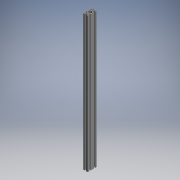
# Autodesk Inventor part: HFS5-2040-600-Z5-YA10-YB590
Saved by Autodesk Inventor 2017.3 (Build 213256000, 256)
## iProperties
Part Number: HFS5-2040-600-Z5-YA10-YB590
Material: Generic
Catalog Web Link: www.cadenas.de
Description: NFS5-2040, NFSB5-2040, HFS5-2040, HFSB5-2040, CAF5-2040, NFSF5-2040, HFSF5-2040-HFS5 Series Aluminum Extrusions 20,40 Square -2 Slots-
Vendor: MISUMI
Document SubType Name: Modeling
Designer: partserver
Manufacturer: MISUMI
Mass: 193.574 g
Surface Area: 1890.72 cm^2
Volume: 193.574 cm^3
Density: 1 g/cm^3
Appearance: PSOLRGB-175-175-175
Category: PARTsolutions
Company: MISUMI
Title: HFS5-2040-600-Z5-YA10-YB590
Author: Cadenas PARTsolutions
Comments: HFS5 Series Aluminum Extrusions 20,40 Square -2 Slots-
PSOL_IDENT_0: {$CADENAS_DATA\23d-libs\misumi\metric\38_al_extrusions_blackets\5\hfs5_2040.prj},643 {VTYP=3D},{NB=H
PSOL_IDENT_1: FS5-2040-600-Z5-YA10-YB590},{LINA=HFS5-2040-600-Z5-YA10-YB590},{NN=NFS5-2040, NFSB5-2040, HFS5-2040,
PSOL_IDENT_2: HFSB5-2040, CAF5-2040, NFSF5-2040, HFSF5-2040},{DATE=09.09.2019 15:28:27},{GEOMDATE=28.10.2014 00:0
PSOL_IDENT_3: 0:00},{VERSION=},{LINEID=150},{WBVAR=L,ALT1,ALT2,ALT4,ALT5,CP5,DL5,DR5,ALT6,ALT9,ALT10,ALT11,HP6,NHL
PSOL_IDENT_4: 6,DL6,NHR6,DR6,ALT7,ALT8,NH9,AH,BH,CH,DH,EH,NH10,AV,BV,CV,DV,EV,NH11,AP,BP,CP,DP,EP,ALT12,ALT13,Z,NH
PSOL_IDENT_5: 12,XA,XB,XC,XD,XE,NH13,YA,YB,YC,YD,YE,ALT16,HP16,DL16,DR16,ALT17,HQ17,JLP,ALT18,HQ18,KLP,ALT20},{WBN
PSOL_IDENT_6: UMERIC=L,NH9,AH,BH,CH,DH,EH,NH10,AV,BV,CV,DV,EV,NH11,AP,BP,CP,DP,EP,NH12,XA,XB,XC,XD,XE,NH13,YA,YB,Y
PSOL_IDENT_7: C,YD,YE,HQ17,JLP,HQ18,KLP}  {NB=HFS5-2040-600-Z5-YA10-YB590},{LINA=HFS5-2040-600-Z5-YA10-YB590},{KT=
PSOL_IDENT_8: DUMMY},{PN=HFS5-2040-600-Z5-YA10-YB590},{TPS=HFS5-2040},{MAT=A6N01SS-T5 Aluminum Alloy},{ST=Clear An
PSOL_IDENT_9: odize},{FRMW=20},{FRMH=40},{FRD=4.2},{L=600},{MASS=0.88},{SA=324},{LX=1.358x10^4},{LY=5.13x10^4},{AL
PSOL_IDENT_10: T1=},{M1=0},{DPL1=0},{DPR1=0},{ALT1PN=},{ALT2=},{ALT2ALG= '','w/o End Tapping (Heli-Coil Insert)','L
PSOL_IDENT_11: HP','with LHP (Tapping on the Left (Heli-Coil Insert))','RHP','with RHP (Tapping on the Right (Heli-
PSOL_IDENT_12: Coil Insert))','HPW','with HPW (Tapping on Both Ends (Heli-Coil Insert))' },{M2=0},{DP2=0},{ALT2PN=}
PSOL_IDENT_13: ,{ALT4=},{ALT4ALG= '', 'w/o SC (High Precision Cut)', 'SC', 'with SC (High Precision Cut)' },{ALT4PN=
PSOL_IDENT_14: },{ALT5=},{ALT5ALG= '','w/o 45 Degree Cut','1','with 45 Degree Cut' },{CP5=},{CP5ALG= '','N/A' },{DL
PSOL_IDENT_15: 5=},{DL5ALG= '','N/A' },{DR5=},{DR5ALG= '','N/A' },{FRMLALT5=0},{FRMRALT5=0},{ALT5PN=},{ALT6=},{ALT6
PSOL_IDENT_16: ALG= '','w/o Fastening Location Wrench Access Hole Alterations','1','with Fastening Location Wrench
PSOL_IDENT_17: Access Hole Alterations' },{ALT9=},{ALT9ALG= '','w/o Location Specified Wrench Access Hole Alteraton
PSOL_IDENT_18: s (Horizontal)','1','with Location Specified Wrench Access Hole Alteratons (Horizontal)' },{ALT10=},
PSOL_IDENT_19: {ALT10ALG= '','w/o Location Specified Wrench Access Hole Alteratons (Vertical)','1','with Location S
PSOL_IDENT_20: pecified Wrench Access Hole Alteratons (Vertical)' },{ALT11=},{ALT11ALG= '','w/o Location Specified
PSOL_IDENT_21: Wrench Access Hole Alteratons (Crisscross)','1','with Location Specified Wrench Access Hole Alterato
PSOL_IDENT_22: ns (Crisscross)' },{HP6=},{HP6ALG= '','N/A' },{NHL6=},{NHL6ALG= '','N/A' },{DL6=},{DL6ALG= '','N/A'
PSOL_IDENT_23: },{NHR6=},{NHR6ALG= '','N/A' },{DR6=},{DR6ALG= '','N/A' },{HL6=0},{HL6D=0},{HR6=0},{HR6D=0},{J6=0},{
PSOL_IDENT_24: J6D=0},{K6=0},{K6D=0},{DD6=0.00},{DD6ALG=0},{ALT7=},{ALT7ALG= '','N/A' },{ALT8=},{ALT8ALG= '','N/A'
PSOL_IDENT_25: },{ALT678PN=},{NH9=0},{NH9MAX=5},{NH9ALG=[0]},{AH=0.0},{AHMIN=7},{AHMAX=595},{AHALG=[0]},{BH=0.0},{B
PSOL_IDENT_26: HMIN=2},{BHMAX=597},{BHALG=[0]},{CH=0.0},{CHMIN=2},{CHMAX=599},{CHALG=[0]},{DH=0.0},{DHMIN=2},{DHMAX=
PSOL_IDENT_27: 601},{DHALG=[0]},{EH=0.0},{EHMIN=2},{EHMAX=593},{EHALG=[0]},{NH10=0},{NH10MAX=5},{NH10ALG=[0]},{AV=0
PSOL_IDENT_28: .0},{AVMIN=7},{AVMAX=595},{AVALG=[0]},{BV=0.0},{BVMIN=2},{BVMAX=597},{BVALG=[0]},{CV=0.0},{CVMIN=2},
PSOL_IDENT_29: {CVMAX=599},{CVALG=[0]},{DV=0.0},{DVMIN=2},{DVMAX=601},{DVALG=[0]},{EV=0.0},{EVMIN=2},{EVMAX=593},{E
PSOL_IDENT_30: VALG=[0]},{NH11=0},{NH11MAX=5},{NH11ALG=[0]},{AP=0.0},{APMIN=7},{APMAX=595},{APALG=[0]},{BP=0.0},{BP
PSOL_IDENT_31: MIN=2},{BPMAX=597},{BPALG=[0]},{CP=0.0},{CPMIN=2},{CPMAX=599},{CPALG=[0]},{DP=0.0},{DPMIN=2},{DPMAX=
PSOL_IDENT_32: 601},{DPALG=[0]},{EP=0.0},{EPMIN=2},{EPMAX=593},{EPALG=[0]},{ALT9PN=},{ALT10PN=},{ALT11PN=},{ALT9101
PSOL_IDENT_33: 1PN=},{ALT12=},{ALT12ALG= '','w/o Counterbore Hole in Specified Position (Vertical)','1','with Count
PSOL_IDENT_34: erbore Hole in Specified Position (Vertical)' },{ALT13=1},{ALT13ALG= '','w/o Counterbore Hole in Spe
PSOL_IDENT_35: cified Position (Horizontal)','1','with Counterbore Hole in Specified Position (Horizontal)' },{Z=5}
PSOL_IDENT_36: ,{ZALG='5','5','6','6'},{DD12=5.5},{DD112=9.5},{NH12=0},{NH12MAX=5},{NH12ALG=[0]},{XA=0.0},{XAMIN=7}
PSOL_IDENT_37: ,{XAMAX=604.5},{XAALG=[0]},{XB=0.0},{XBMIN=11.5},{XBMAX=616},{XBALG=[0]},{XC=0.0},{XCMIN=11.5},{XCMA
PSOL_IDENT_38: X=627.5},{XCALG=[0]},{XD=0.0},{XDMIN=11.5},{XDMAX=639},{XDALG=[0]},{XE=0.0},{XEMIN=11.5},{XEMAX=593}
PSOL_IDENT_39: ,{XEALG=[0]},{NH13=2},{NH13MAX=5},{NH13ALG=[1:5/1]},{YA=10.0},{YAMIN=7},{YAMAX=581.5},{YAALG=[7:581.
PSOL_IDENT_40: 5/0.5]},{YB=590.0},{YBMIN=21.5},{YBMAX=593},{YBALG=[21.5:593/0.5]},{YC=0.0},{YCMIN=601.5},{YCMAX=604
PSOL_IDENT_41: .5},{YCALG=[0]},{YD=0.0},{YDMIN=11.5},{YDMAX=616},{YDALG=[0]},{YE=0.0},{YEMIN=11.5},{YEMAX=593},{YEA
PSOL_IDENT_42: LG=[0]},{ALT12PN=},{ALT13PN=-YA10-YB590},{ALT1213PN=-Z5-YA10-YB590},{ALT16=},{ALT16ALG= '','w/o M Ty
PSOL_IDENT_43: pe Hole Alteration','1','with M Type Hole Alteration' },{HP16=},{HP16ALG= '','N/A' },{DL16=},{DL16AL
PSOL_IDENT_44: G= '','N/A' },{DR16=},{DR16ALG= '','N/A' },{H116=0},{D16=0.0},{ALT16PN=},{ALT17=},{ALT17ALG= '','w/o
PSOL_IDENT_45: L Type Hole Alteration (Top)','1','with L Type Hole Alteration (Top)' },{HQ17=0},{HQ17ALG=0},{JLP=0
PSOL_IDENT_46: },{JLPMIN=4.9},{JLPMAX=0},{JLPALG=[0]},{L17=0},{D17=0.0},{ALT18=},{ALT18ALG= '','w/o L Type Hole Alt
PSOL_IDENT_47: eration (Bottom)','1','with L Type Hole Alteration (Bottom)' },{HQ18=0},{HQ18ALG=0},{KLP=0},{KLPMIN=
PSOL_IDENT_48: 4.9},{KLPMAX=0},{KLPALG=[0]},{L18=0},{D18=0.0},{ALT1718PN=},{ALT20=},{ALT20PN=},{ERRORALT01=OK},{ERR
PSOL_IDENT_49: ORALT02=OK},{ERRORALT05=OK},{ERRORALT06091=OK},{ERRORALT06092=OK},{ERRORALT06093=OK},{ERRORALT06094=
PSOL_IDENT_50: OK},{ERRORALT06101=OK},{ERRORALT06102=OK},{ERRORALT06103=OK},{ERRORALT06104=OK},{ERRORALT06111=OK},{
PSOL_IDENT_51: ERRORALT06112=OK},{ERRORALT06113=OK},{ERRORALT06114=OK},{ERRORALT06121=OK},{ERRORALT06122=OK},{ERROR
PSOL_IDENT_52: ALT06123=OK},{ERRORALT06124=OK},{ERRORALT06131=OK},{ERRORALT06132=OK},{ERRORALT06133=OK},{ERRORALT06
PSOL_IDENT_53: 134=OK},{ERRORALT0616=OK},{ERRORALT06171=OK},{ERRORALT06172=OK},{ERRORALT06173=OK},{ERRORALT06181=OK
PSOL_IDENT_54: },{ERRORALT06182=OK},{ERRORALT06183=OK},{ERRORALT0911=OK},{ERRORALT0913=OK},{ERRORALT0916=OK},{ERROR
PSOL_IDENT_55: ALT0917=OK},{ERRORALT0918=OK},{ERRORALT1011=OK},{ERRORALT1012=OK},{ERRORALT1016=OK},{ERRORALT1017=OK
PSOL_IDENT_56: },{ERRORALT1018=OK},{ERRORALT1112=OK},{ERRORALT1113=OK},{ERRORALT1116=OK},{ERRORALT1117=OK},{ERRORAL
PSOL_IDENT_57: T1118=OK},{ERRORALT1216=OK},{ERRORALT1217=OK},{ERRORALT1218=OK},{ERRORALT1316=OK},{ERRORALT1317=OK},
PSOL_IDENT_58: {ERRORALT1318=OK},{ERRORALT1617=OK},{ERRORALT1618=OK},{ERRORPN=},{TFW=0}
NB: HFS5-2040-600-Z5-YA10-YB590
NN: NFS5-2040, NFSB5-2040, HFS5-2040, HFSB5-2040, CAF5-2040, NFSF5-2040, HFSF5-2040
NT: HFS5 Series Aluminum Extrusions 20,40 Square -2 Slots-
NBSYN: $PN.
LINA: HFS5-2040-600-Z5-YA10-YB590
CATALOG: Misumi
PN: HFS5-2040-600-Z5-YA10-YB590
TPS: HFS5-2040
MAT: A6N01SS-T5 Aluminum Alloy
ST: Clear Anodize
L: 600
MASS: 0.88
SA: 324
LX: 1.358x10^4
LY: 5.13x10^4
ALT1: w/o End Tapping
M1: 0
DPL1: 0
DPR1: 0
ALT2: w/o End Tapping (Heli-Coil Insert)
M2: 0
DP2: 0
ALT4: w/o SC (High Precision Cut)
ALT5: w/o 45 Degree Cut
CP5: N/A
DL5: N/A
DR5: N/A
ALT6: w/o Fastening Location Wrench Access Hole Alterations
ALT9: w/o Location Specified Wrench Access Hole Alteratons (Horizontal)
ALT10: w/o Location Specified Wrench Access Hole Alteratons (Vertical)
ALT11: w/o Location Specified Wrench Access Hole Alteratons (Crisscross)
HP6: N/A
NHL6: N/A
DL6: N/A
NHR6: N/A
DR6: N/A
HL6D: 0
HR6D: 0
J6D: 0
K6D: 0
DD6: 0
ALT7: N/A
ALT8: N/A
NH9: 0
AH: 0
BH: 0
CH: 0
DH: 0
EH: 0
NH10: 0
AV: 0
BV: 0
CV: 0
DV: 0
EV: 0
NH11: 0
AP: 0
BP: 0
CP: 0
DP: 0
EP: 0
ALT12: w/o Counterbore Hole in Specified Position (Vertical)
ALT13: with Counterbore Hole in Specified Position (Horizontal)
Z: 5
DD12: 5.5
DD112: 9.5
NH12: 0
XA: 0
XB: 0
XC: 0
XD: 0
XE: 0
NH13: 2
YA: 10
YB: 590
YC: 0
YD: 0
YE: 0
ALT16: w/o M Type Hole Alteration
HP16: N/A
DL16: N/A
DR16: N/A
H116: 0
D16: 0
ALT17: w/o L Type Hole Alteration (Top)
HQ17: 0
JLP: 0
D17: 0
ALT18: w/o L Type Hole Alteration (Bottom)
HQ18: 0
KLP: 0
D18: 0
ALT20: w/o CW (End Face C Chamfering)
SUPPLIER: MISUMI
ARTICLENO: HFS5-2040-600-Z5-YA10-YB590
BOMINFO: HFS5-2040-600-Z5-YA10-YB590
CREATOR: CADENAS GmbH
Autodesk Inventor part; units mm, degrees
ref_plane "YZ Plane" through (0, 0, 0) normal (1, 0, 0) x (0, 1, 0)
ref_plane "XZ Plane" through (0, 0, 0) normal (0, 1, 0) x (-1, 0, 0)
ref_plane "XY Plane" through (0, 0, 0) normal (0, 0, 1) x (1, 0, 0)
sketch "Sketch_1" plane through (0, 0, 0) normal (0, 0, 1) x (1, 0, 0)
  line L0 (-10, -7) -> (-8, -7)
  line L1 (-8, -7) -> (-8, -4)
  line L2 (-8, -4) -> (-7.0607, -4)
  line L3 (-7.0607, -4) -> (-4, -7.0607)
  line L4 (-4, -7.0607) -> (-4, -9.4804)
  line L5 (-4, -9.4804) -> (-3.7, -10)
  line L6 (-3.7, -10) -> (-4, -10.5196)
  line L7 (-4, -10.5196) -> (-4, -12.9393)
  line L8 (-4, -12.9393) -> (-7.0607, -16)
  line L9 (-7.0607, -16) -> (-8, -16)
  line L10 (-8, -16) -> (-8, -13)
  line L11 (-8, -13) -> (-10, -13)
  line L12 (-10, -13) -> (-10, -19)
  arc A0 (-10, -19) -> (-9, -20) centre (-9, -19) ccw
  line L13 (-9, -20) -> (-3, -20)
  line L14 (-3, -20) -> (-3, -18)
  line L15 (-3, -18) -> (-6, -18)
  line L16 (-6, -18) -> (-6, -17.0607)
  line L17 (-6, -17.0607) -> (-2.9393, -14)
  line L18 (-2.9393, -14) -> (-0.5196, -14)
  line L19 (-0.5196, -14) -> (0, -13.7)
  line L20 (0, -13.7) -> (0.5196, -14)
  line L21 (0.5196, -14) -> (2.9393, -14)
  line L22 (2.9393, -14) -> (6, -17.0607)
  line L23 (6, -17.0607) -> (6, -18)
  line L24 (6, -18) -> (3, -18)
  line L25 (3, -18) -> (3, -20)
  line L26 (3, -20) -> (9, -20)
  arc A1 (9, -20) -> (10, -19) centre (9, -19) ccw
  line L27 (10, -19) -> (10, -13)
  line L28 (10, -13) -> (8, -13)
  line L29 (8, -13) -> (8, -16)
  line L30 (8, -16) -> (7.0607, -16)
  line L31 (7.0607, -16) -> (4, -12.9393)
  line L32 (4, -12.9393) -> (4, -10.5196)
  line L33 (4, -10.5196) -> (3.7, -10)
  line L34 (3.7, -10) -> (4, -9.4804)
  line L35 (4, -9.4804) -> (4, -7.0607)
  line L36 (4, -7.0607) -> (7.0607, -4)
  line L37 (7.0607, -4) -> (8, -4)
  line L38 (8, -4) -> (8, -7)
  line L39 (8, -7) -> (10, -7)
  line L40 (10, -7) -> (10, 7)
  line L41 (10, 7) -> (8, 7)
  line L42 (8, 7) -> (8, 4)
  line L43 (8, 4) -> (7.0607, 4)
  line L44 (7.0607, 4) -> (4, 7.0607)
  line L45 (4, 7.0607) -> (4, 9.4804)
  line L46 (4, 9.4804) -> (3.7, 10)
  line L47 (3.7, 10) -> (4, 10.5196)
  line L48 (4, 10.5196) -> (4, 12.9393)
  line L49 (4, 12.9393) -> (7.0607, 16)
  line L50 (7.0607, 16) -> (8, 16)
  line L51 (8, 16) -> (8, 13)
  line L52 (8, 13) -> (10, 13)
  line L53 (10, 13) -> (10, 19)
  arc A2 (10, 19) -> (9, 20) centre (9, 19) ccw
  line L54 (9, 20) -> (3, 20)
  line L55 (3, 20) -> (3, 18)
  line L56 (3, 18) -> (6, 18)
  line L57 (6, 18) -> (6, 17.0607)
  line L58 (6, 17.0607) -> (2.9393, 14)
  line L59 (2.9393, 14) -> (0.5196, 14)
  line L60 (0.5196, 14) -> (0, 13.7)
  line L61 (0, 13.7) -> (-0.5196, 14)
  line L62 (-0.5196, 14) -> (-2.9393, 14)
  line L63 (-2.9393, 14) -> (-6, 17.0607)
  line L64 (-6, 17.0607) -> (-6, 18)
  line L65 (-6, 18) -> (-3, 18)
  line L66 (-3, 18) -> (-3, 20)
  line L67 (-3, 20) -> (-9, 20)
  arc A3 (-9, 20) -> (-10, 19) centre (-9, 19) ccw
  line L68 (-10, 19) -> (-10, 13)
  line L69 (-10, 13) -> (-8, 13)
  line L70 (-8, 13) -> (-8, 16)
  line L71 (-8, 16) -> (-7.0607, 16)
  line L72 (-7.0607, 16) -> (-4, 12.9393)
  line L73 (-4, 12.9393) -> (-4, 10.5196)
  line L74 (-4, 10.5196) -> (-3.7, 10)
  line L75 (-3.7, 10) -> (-4, 9.4804)
  line L76 (-4, 9.4804) -> (-4, 7.0607)
  line L77 (-4, 7.0607) -> (-7.0607, 4)
  line L78 (-7.0607, 4) -> (-8, 4)
  line L79 (-8, 4) -> (-8, 7)
  line L80 (-8, 7) -> (-10, 7)
  line L81 (-10, 7) -> (-10, -7)
  line L82 (-8, 1.7) -> (-8, -1.7)
  arc A4 (-8, -1.7) -> (-7.7, -2) centre (-7.7, -1.7) ccw
  line L83 (-7.7, -2) -> (-7.0636, -2)
  arc A5 (-6.8515, -2.0879) -> (-7.0636, -2) centre (-7.0636, -2.3) ccw
  line L84 (-6.8515, -2.0879) -> (-2.9393, -6)
  line L85 (-2.9393, -6) -> (2.9393, -6)
  line L86 (2.9393, -6) -> (6.8515, -2.0879)
  arc A6 (7.0636, -2) -> (6.8515, -2.0879) centre (7.0636, -2.3) ccw
  line L87 (7.0636, -2) -> (7.7, -2)
  arc A7 (7.7, -2) -> (8, -1.7) centre (7.7, -1.7) ccw
  line L88 (8, -1.7) -> (8, 1.7)
  arc A8 (8, 1.7) -> (7.7, 2) centre (7.7, 1.7) ccw
  line L89 (7.7, 2) -> (7.0636, 2)
  arc A9 (6.8515, 2.0879) -> (7.0636, 2) centre (7.0636, 2.3) ccw
  line L90 (6.8515, 2.0879) -> (2.9393, 6)
  line L91 (2.9393, 6) -> (-2.9393, 6)
  line L92 (-2.9393, 6) -> (-6.8515, 2.0879)
  arc A10 (-7.0636, 2) -> (-6.8515, 2.0879) centre (-7.0636, 2.3) ccw
  line L93 (-7.0636, 2) -> (-7.7, 2)
  arc A11 (-7.7, 2) -> (-8, 1.7) centre (-7.7, 1.7) ccw
  constraints: 188 end point, 24 point on circle, 12 centre point
extrude "Extrusion1" add sketch "Sketch_1" against normal blind 600
sketch "Sketch2" plane through (0, 0, -600) normal (0, 0, -1) x (-1, 0, 0)
  point P0 (0, 10)
hole "Hole1" at (0, 10, -600) direction (0, 0, 1) diameter 4.2 depth 600
pattern_linear "Rectangular Pattern1" count 2 spacing 20 along (0, -1, 0) of "Hole1"
sketch "Sketch_50" plane through (0, 10, 0) normal (0, 1, 0) x (1, 0, 0)
  line L0 (10, 10) -> (-10, 10)
  line L1 (-10, 10) -> (-10, 12.75)
  line L2 (-10, 12.75) -> (4, 12.75)
  line L3 (4, 12.75) -> (4, 14.75)
  line L4 (4, 14.75) -> (10, 14.75)
  line L5 (10, 14.75) -> (10, 10)
  line L6 (10, 10) -> (-10, 10)
  constraints: 14 end point
revolve "Revolution1" cut sketch "Sketch_50" angle 360 about axis through (10, 10, -10) along (1, 0, 0)
sketch "_p_______27_Sketch_50_0" plane through (0, -10, 0) normal (0, 1, 0) x (1, 0, 0)
  line L0 (10, 10) -> (-10, 10)
  line L1 (-10, 10) -> (-10, 12.75)
  line L2 (-10, 12.75) -> (4, 12.75)
  line L3 (4, 12.75) -> (4, 14.75)
  line L4 (4, 14.75) -> (10, 14.75)
  line L5 (10, 14.75) -> (10, 10)
  line L6 (10, 10) -> (-10, 10)
  constraints: 14 end point
revolve "Revolution2" cut sketch "_p_______27_Sketch_50_0" angle 360 about axis through (10, -10, -10) along (1, 0, 0)
sketch "Sketch_51" plane through (0, 10, 0) normal (0, 1, 0) x (1, 0, 0)
  line L0 (10, 590) -> (-10, 590)
  line L1 (-10, 590) -> (-10, 592.75)
  line L2 (-10, 592.75) -> (4, 592.75)
  line L3 (4, 592.75) -> (4, 594.75)
  line L4 (4, 594.75) -> (10, 594.75)
  line L5 (10, 594.75) -> (10, 590)
  line L6 (10, 590) -> (-10, 590)
  constraints: 14 end point
revolve "Revolution3" cut sketch "Sketch_51" angle 360 about axis through (10, 10, -590) along (1, 0, 0)
sketch "_p_______28_Sketch_51_0" plane through (0, -10, 0) normal (0, 1, 0) x (1, 0, 0)
  line L0 (10, 590) -> (-10, 590)
  line L1 (-10, 590) -> (-10, 592.75)
  line L2 (-10, 592.75) -> (4, 592.75)
  line L3 (4, 592.75) -> (4, 594.75)
  line L4 (4, 594.75) -> (10, 594.75)
  line L5 (10, 594.75) -> (10, 590)
  line L6 (10, 590) -> (-10, 590)
  constraints: 14 end point
revolve "Revolution4" cut sketch "_p_______28_Sketch_51_0" angle 360 about axis through (10, -10, -590) along (1, 0, 0)
ref_plane "C1_XY" through (0, 0, 0) normal (0, 0, 1) x (1, 0, 0)
ref_plane "C1_YZ" through (0, 0, 0) normal (1, 0, 0) x (0, 1, 0)
ref_plane "C1_ZX" through (0, 0, 0) normal (0, 1, 0) x (0, 0, 1)
body "Solid1"
